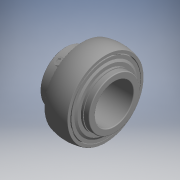
# Autodesk Inventor part: YAR 206-2RF-39.710300320618 -bearing
Saved by Autodesk Inventor 2017.3 (Build 213256000, 256)
## iProperties
Part Number: YAR 206-2RF-39.710300320618 -bearing
Material: Generic
Catalog Web Link: www.cadenas.de
Description: ayf_001hc_hh_hy_bearing-Y-bearings
Vendor: SKF
Document SubType Name: Modeling
Designer: partserver
Manufacturer: SKF
Mass: 35.182 g
Surface Area: 305.499 cm^2
Volume: 35.182 cm^3
Density: 1 g/cm^3
Appearance: PSOLRGB-175-175-175
Category: PARTsolutions
Company: SKF
Title: YAR 206-2RF-39.710300320618 -bearing
Author: Cadenas PARTsolutions
Comments: Y-bearings
PSOL_IDENT_0: {$CADENAS_DATA\23d-libs\skf\bearings_units_and_housings\bearing_units\ball_bearing_units\y-units\y-b
PSOL_IDENT_1: earing_square_flanged_units_parts\ayf_001hc_hh_hy_bearing.prj},231 {VTYP=3D},{NB=YAR 206-2RF-39.7103
PSOL_IDENT_2: 00320618 -bearing},{LINA=YAR 206-2RF-39.710300320618 -bearing},{NN=ayf_001hc_hh_hy_bearing},{DATE=20
PSOL_IDENT_3: .08.2020 13:45:20},{GEOMDATE=29.07.2020 17:09:33},{VERSION=},{LINEID=1120},{WBVAR=},{WBNUMERIC=}  {N
PSOL_IDENT_4: B=YAR 206-2RF-39.710300320618 -bearing},{LINA=YAR 206-2RF-39.710300320618 -bearing},{KT=DUMMY},{PROD
PSOL_IDENT_5: UCTID=103003206},{DESIGNATION=YAR 206-2RF},{DD=30.0000},{D=62},{B=38.100},{C=18.000},{PITCH=46.000},
PSOL_IDENT_6: {DW=9.525},{FO=IEC_BBY_006},{DESIGN=ybrg1},{B1=MIN},{LM=Grub screw},{DES=Inner ring extended on both
PSOL_IDENT_7: sides},{PS=For agricultural applications},{MAT=},{SS=Multiple seals},{UNIT=Metric},{G=MIN},{DD1=39.
PSOL_IDENT_8: 70},{DD2=MIN},{DD3=MIN},{B3=0.000},{B4=MIN},{BB4=5.0},{R12=0.6},{R12X=0},{SS1=22.200},{NOTE=},{DG=MI
PSOL_IDENT_9: N},{E=5.100},{F=1.700},{RG=MIN},{LOAD1=19.500},{LOAD2=11.200},{LOAD3=0.475},{SPEED2=3800},{FF0=14},{
PSOL_IDENT_10: BF=1},{A15=500000},{A8=400000},{A4=300000},{BETA=1.62},{SBT1=0.415},{SBT2=},{RF1=0.00000039},{RF2=1.
PSOL_IDENT_11: 7},{SF1=0.00323},{SF2=36.5},{KZ=3.1},{II=1},{Z=9},{SG=VT307},{MASS=0.31},{G2=M6x0.75},{HEX=3.000},{R
PSOL_IDENT_12: TT=4},{MKIT=},{AS=},{TANGLE=},{SLEEVE=},{SRING=RIS 206 A},{FPC=RBC17_YBRG_001},{POPI=1},{NOUN=N020},
PSOL_IDENT_13: {NOUNDES=Ball bearing},{MOD=M200},{MODDES=Radial deep groove},{YZ=19.85},{PIM=YAR 206-2RF},{LNDD11=M
PSOL_IDENT_14: IN},{LUB3=0},{BZ=0.565},{SDALG=h},{YRZ=27.7625},{SHAPE=5},{LNB1HM11=0},{LWM=0},{TYPEID=103003},{LUBG
PSOL_IDENT_15: R2=0},{LOCKNUT=},{LOCKDEVICE=},{LNB=MIN},{BB=MIN},{LNB1=MIN},{S1ALG=22.2},{HH=MIN},{LDB=MIN},{LDDD1=
PSOL_IDENT_16: MIN},{LDDD2=MIN},{LDM=MIN},{LDFF=MIN},{TP=4},{LNBHM11=0},{BBHM11=0},{LNDD1HM11=0},{HELP=5},{HHHM11=0
PSOL_IDENT_17: },{LUBGR1=0},{LWV=0},{S2=28.5},{LUB2=1},{BZ1=0.000},{HEX2=}
NB: YAR 206-2RF-39.710300320618 -bearing
NN: ayf_001hc_hh_hy_bearing
NT: Y-bearings
NBSYN: $DESIGNATION.-$DD1.$PRODUCTID.$C.$B1.-bearing
LINA: YAR 206-2RF-39.710300320618 -bearing
CATALOG: SKF
DESIGNATION: YAR 206-2RF
DD: 30
D: 62
B: 38.1
C: 18
B1: 0
DD1: 39.7
LOAD1: 19.5
LOAD2: 11.2
LOAD3: 0.475
SPEED2: 3800
SUPPLIER: SKF
ARTICLENO: YAR 206-2RF-39.710300320618 -bearing
BOMINFO: YAR 206-2RF-39.710300320618 -bearing
CREATOR: CADENAS GmbH
Autodesk Inventor part; units mm, degrees
sketch "Sketch_1" plane through (0, 0, 0) normal (0, 0, 1) x (1, 0, 0)
  line L0 (50, 0) -> (-50, 0)
  arc A0 (-15.9, 15.6) -> (-15.3, 15) centre (-15.3, 15.6) ccw
  line L1 (-15.3, 15) -> (21.6, 15)
  arc A1 (21.6, 15) -> (22.2, 15.6) centre (21.6, 15.6) ccw
  line L2 (22.2, 15.6) -> (22.2, 19.25)
  arc A2 (22.2, 19.25) -> (21.6, 19.85) centre (21.6, 19.25) ccw
  line L3 (21.6, 19.85) -> (3.572, 19.85)
  arc A3 (-3.572, 19.85) -> (3.572, 19.85) centre (0, 23) ccw
  line L4 (-3.572, 19.85) -> (-15.3, 19.85)
  arc A4 (-15.3, 19.85) -> (-15.9, 19.25) centre (-15.3, 19.25) ccw
  line L5 (-15.9, 19.25) -> (-15.9, 15.6)
  constraints: 12 end point, 10 point on circle, 5 centre point
revolve "Revolution1" add sketch "Sketch_1" angle 360 about axis through (50, 0, 0) along (1, 0, 0)
sketch "Sketch_2" plane through (0, 15, 0) normal (0, 1, 0) x (1, 0, 0)
  circle A0 centre (17.2, 0) radius 3
  line L0 (15.7, -0.866) -> (17.2, -1.7321)
  line L1 (17.2, -1.7321) -> (18.7, -0.866)
  line L2 (18.7, -0.866) -> (18.7, 0.866)
  line L3 (18.7, 0.866) -> (17.2, 1.7321)
  line L4 (17.2, 1.7321) -> (15.7, 0.866)
  line L5 (15.7, 0.866) -> (15.7, -0.866)
  constraints: 12 end point, 1 centre point
extrude "Extrusion1" add sketch "Sketch_2" along normal blind 5.335
sketch "Sketch_3" plane through (0, -7.5, -12.9904) normal (0, -0.5, -0.866) x (1, 0, 0)
  circle A0 centre (17.2, 0) radius 3
  line L0 (15.7, -0.866) -> (17.2, -1.7321)
  line L1 (17.2, -1.7321) -> (18.7, -0.866)
  line L2 (18.7, -0.866) -> (18.7, 0.866)
  line L3 (18.7, 0.866) -> (17.2, 1.7321)
  line L4 (17.2, 1.7321) -> (15.7, 0.866)
  line L5 (15.7, 0.866) -> (15.7, -0.866)
  constraints: 12 end point, 1 centre point
extrude "Extrusion2" add sketch "Sketch_3" along normal blind 5.335
sketch "Sketch_10" plane through (0, 0, 0) normal (0, 0, 1) x (1, 0, 0)
  line L0 (9, 0) -> (-9, 0)
  line L1 (-11.8525, 20.415) -> (-11.8525, 19.85)
  line L2 (-11.8525, 19.85) -> (-9.5925, 19.85)
  line L3 (-9.5925, 19.85) -> (-9.5925, 22.4564)
  arc A0 (-9.1678, 23.3393) -> (-9.5925, 22.4564) centre (-8.4625, 22.4564) ccw
  line L4 (-9.1678, 23.3393) -> (-8.435, 23.9246)
  line L5 (-8.435, 23.9246) -> (-8.435, 20.3248)
  line L6 (-8.435, 20.3248) -> (-7.87, 20.3248)
  line L7 (-7.87, 20.3248) -> (-7.87, 23.6289)
  line L8 (-7.87, 23.6289) -> (-6.0852, 24.8663)
  line L9 (-6.0852, 24.8663) -> (-6.0209, 24.7734)
  line L10 (-6.0209, 24.7734) -> (-7.757, 23.5697)
  line L11 (-7.757, 23.5697) -> (-7.757, 20.5621)
  line L12 (-7.757, 20.5621) -> (-6.1938, 20.5621)
  line L13 (-6.1938, 20.5621) -> (-6.3633, 19.85)
  line L14 (-6.3633, 19.85) -> (-5.7983, 19.85)
  line L15 (-5.7983, 19.85) -> (-5.61, 20.6413)
  line L16 (-5.61, 20.6413) -> (-5.61, 21.4325)
  line L17 (-5.61, 21.4325) -> (-6.3633, 22.2237)
  line L18 (-6.3633, 22.2237) -> (-6.3633, 23.8062)
  line L19 (-6.3633, 23.8062) -> (-5.61, 24.5975)
  line L20 (-5.61, 24.5975) -> (-5.61, 27.5742)
  arc A1 (-5.61, 27.5742) -> (-5.7983, 27.7625) centre (-5.7983, 27.5742) ccw
  line L21 (-5.7983, 27.7625) -> (-5.9867, 27.7625)
  arc A2 (-5.9867, 27.7625) -> (-6.175, 27.5742) centre (-5.9867, 27.5742) ccw
  line L22 (-6.175, 27.5742) -> (-7.1728, 26.385)
  line L23 (-7.1728, 26.385) -> (-6.74, 26.0218)
  line L24 (-6.74, 26.0218) -> (-6.175, 26.6952)
  line L25 (-6.175, 26.6952) -> (-6.175, 25.4916)
  line L26 (-6.175, 25.4916) -> (-7.6697, 24.4552)
  line L27 (-7.6697, 24.4552) -> (-8.7175, 24.5875)
  line L28 (-8.7175, 24.5875) -> (-8.7175, 26.98)
  line L29 (-8.7175, 26.98) -> (-9.2825, 26.98)
  line L30 (-9.2825, 26.98) -> (-9.2825, 24.5875)
  line L31 (-9.2825, 24.5875) -> (-10.1575, 23)
  line L32 (-10.1575, 23) -> (-10.1575, 20.415)
  line L33 (-10.1575, 20.415) -> (-11.8525, 20.415)
  constraints: 68 end point, 6 point on circle, 3 centre point
sketch "Sketch_15" plane through (0, 0, 0) normal (0, 0, 1) x (1, 0, 0)
  line L0 (9, 0) -> (-9, 0)
  line L1 (5.61, 27.5742) -> (5.61, 24.5975)
  line L2 (5.61, 24.5975) -> (6.3633, 23.8062)
  line L3 (6.3633, 23.8062) -> (6.3633, 22.2237)
  line L4 (6.3633, 22.2237) -> (5.61, 21.4325)
  line L5 (5.61, 21.4325) -> (5.61, 20.6413)
  line L6 (5.61, 20.6413) -> (5.7983, 19.85)
  line L7 (5.7983, 19.85) -> (6.3633, 19.85)
  line L8 (6.3633, 19.85) -> (6.1938, 20.5621)
  line L9 (6.1938, 20.5621) -> (7.757, 20.5621)
  line L10 (7.757, 20.5621) -> (7.757, 23.5697)
  line L11 (7.757, 23.5697) -> (6.0209, 24.7734)
  line L12 (6.0209, 24.7734) -> (6.0852, 24.8663)
  line L13 (6.0852, 24.8663) -> (7.87, 23.6289)
  line L14 (7.87, 23.6289) -> (7.87, 20.3248)
  line L15 (7.87, 20.3248) -> (8.435, 20.3248)
  line L16 (8.435, 20.3248) -> (8.435, 23.9246)
  line L17 (8.435, 23.9246) -> (9.1678, 23.3393)
  arc A0 (9.5925, 22.4564) -> (9.1678, 23.3393) centre (8.4625, 22.4564) ccw
  line L18 (9.5925, 22.4564) -> (9.5925, 19.85)
  line L19 (9.5925, 19.85) -> (11.8525, 19.85)
  line L20 (11.8525, 19.85) -> (11.8525, 20.415)
  line L21 (11.8525, 20.415) -> (10.1575, 20.415)
  line L22 (10.1575, 20.415) -> (10.1575, 23)
  line L23 (10.1575, 23) -> (9.2825, 24.5875)
  line L24 (9.2825, 24.5875) -> (9.2825, 26.98)
  line L25 (9.2825, 26.98) -> (8.7175, 26.98)
  line L26 (8.7175, 26.98) -> (8.7175, 24.5875)
  line L27 (8.7175, 24.5875) -> (7.6697, 24.4552)
  line L28 (7.6697, 24.4552) -> (6.175, 25.4916)
  line L29 (6.175, 25.4916) -> (6.175, 26.6952)
  line L30 (6.175, 26.6952) -> (6.74, 26.0218)
  line L31 (6.74, 26.0218) -> (7.1728, 26.385)
  line L32 (7.1728, 26.385) -> (6.175, 27.5742)
  arc A1 (6.175, 27.5742) -> (5.9867, 27.7625) centre (5.9867, 27.5742) ccw
  line L33 (5.9867, 27.7625) -> (5.7983, 27.7625)
  arc A2 (5.7983, 27.7625) -> (5.61, 27.5742) centre (5.7983, 27.5742) ccw
  constraints: 68 end point, 6 point on circle, 3 centre point
sketch "Sketch_16" plane through (0, 0, 0) normal (0, 0, 1) x (1, 0, 0)
  line L0 (9, 0) -> (-9, 0)
  line L1 (-9, 27.505) -> (-6.2842, 27.505)
  line L2 (-6.2842, 27.505) -> (-6.0901, 27.6774)
  arc A0 (-5.6026, 27.5218) -> (-6.0901, 27.6774) centre (-5.8925, 27.455) ccw
  line L3 (-5.6026, 27.5218) -> (-5.4743, 26.9651)
  arc A1 (-5.4743, 26.9651) -> (-5.2794, 26.81) centre (-5.2794, 27.01) ccw
  line L4 (-5.2794, 26.81) -> (-2.9409, 26.81)
  arc A2 (-2.9409, 26.81) -> (-2.792, 26.8582) centre (-2.9409, 27.064) ccw
  arc A3 (2.792, 26.8582) -> (-2.792, 26.8582) centre (0, 23) ccw
  arc A4 (2.792, 26.8582) -> (2.9409, 26.81) centre (2.9409, 27.064) ccw
  line L5 (2.9409, 26.81) -> (5.2794, 26.81)
  arc A5 (5.2794, 26.81) -> (5.4743, 26.9651) centre (5.2794, 27.01) ccw
  line L6 (5.4743, 26.9651) -> (5.6026, 27.5218)
  arc A6 (6.0901, 27.6774) -> (5.6026, 27.5218) centre (5.8925, 27.455) ccw
  line L7 (6.0901, 27.6774) -> (6.2842, 27.505)
  line L8 (6.2842, 27.505) -> (9, 27.505)
  line L9 (9, 27.505) -> (9, 29.5161)
  arc A7 (9, 29.5161) -> (8.8571, 29.7078) centre (8.8, 29.5161) ccw
  arc A8 (8.8571, 29.7078) -> (-8.8571, 29.7078) centre (0, 0) ccw
  arc A9 (-8.8571, 29.7078) -> (-9, 29.5161) centre (-8.8, 29.5161) ccw
  line L10 (-9, 29.5161) -> (-9, 27.505)
  constraints: 22 end point, 20 point on circle, 10 centre point
revolve "Revolution2" add sketch "Sketch_15" angle 360 about axis through (9, 0, 0) along (1, 0, 0)
revolve "Revolution3" add sketch "Sketch_16" angle 360 about axis through (9, 0, 0) along (1, 0, 0)
revolve "Revolution4" add sketch "Sketch_10" angle 360 about axis through (9, 0, 0) along (1, 0, 0)
sketch "Sketch_21" plane through (0, 0, 0) normal (0, 0, 1) x (1, 0, 0)
  line L0 (-4.1475, 23) -> (-4.1475, 46)
  line L1 (-4.1475, 46) -> (-3.2975, 46)
  line L2 (-3.2975, 46) -> (-3.2975, 23)
  line L3 (-3.2975, 23) -> (-4.1475, 23)
  line L4 (-4.1475, 23) -> (-4.1475, 46)
  constraints: 10 end point
revolve "Revolution5" cut sketch "Sketch_21" angle 360 about axis through (-4.1475, 23, 0) along (0, -1, 0)
ref_plane "ball_1_XY" through (0, 23, 0) normal (1, 0, 0) x (0, 0, -1)
ref_plane "ball_1_YZ" through (0, 23, 0) normal (0, 0, -1) x (0, 1, 0)
ref_plane "ball_1_ZX" through (0, 23, 0) normal (0, 1, 0) x (1, 0, 0)
ref_plane "ball_2_XY" through (0, 17.619, 14.7841) normal (1, 0, 0) x (0, 0, -1)
ref_plane "ball_2_YZ" through (0, 17.619, 14.7841) normal (0, 0, -1) x (0, 1, 0)
ref_plane "ball_2_ZX" through (0, 17.619, 14.7841) normal (0, 1, 0) x (1, 0, 0)
ref_plane "ball_3_XY" through (0, 3.9939, 22.6506) normal (1, 0, 0) x (0, 0, -1)
ref_plane "ball_3_YZ" through (0, 3.9939, 22.6506) normal (0, 0, -1) x (0, 1, 0)
ref_plane "ball_3_ZX" through (0, 3.9939, 22.6506) normal (0, 1, 0) x (1, 0, 0)
ref_plane "ball_4_XY" through (0, -11.5, 19.9186) normal (1, 0, 0) x (0, 0, -1)
ref_plane "ball_4_YZ" through (0, -11.5, 19.9186) normal (0, 0, -1) x (0, 1, 0)
ref_plane "ball_4_ZX" through (0, -11.5, 19.9186) normal (0, 1, 0) x (1, 0, 0)
ref_plane "ball_5_XY" through (0, -21.6129, 7.8665) normal (1, 0, 0) x (0, 0, -1)
ref_plane "ball_5_YZ" through (0, -21.6129, 7.8665) normal (0, 0, -1) x (0, 1, 0)
ref_plane "ball_5_ZX" through (0, -21.6129, 7.8665) normal (0, 1, 0) x (1, 0, 0)
ref_plane "ball_6_XY" through (0, -21.6129, -7.8665) normal (1, 0, 0) x (0, 0, -1)
ref_plane "ball_6_YZ" through (0, -21.6129, -7.8665) normal (0, 0, -1) x (0, 1, 0)
ref_plane "ball_6_ZX" through (0, -21.6129, -7.8665) normal (0, 1, 0) x (1, 0, 0)
ref_plane "ball_7_XY" through (0, -11.5, -19.9186) normal (1, 0, 0) x (0, 0, -1)
ref_plane "ball_7_YZ" through (0, -11.5, -19.9186) normal (0, 0, -1) x (0, 1, 0)
ref_plane "ball_7_ZX" through (0, -11.5, -19.9186) normal (0, 1, 0) x (1, 0, 0)
ref_plane "ball_8_XY" through (0, 3.9939, -22.6506) normal (1, 0, 0) x (0, 0, -1)
ref_plane "ball_8_YZ" through (0, 3.9939, -22.6506) normal (0, 0, -1) x (0, 1, 0)
ref_plane "ball_8_ZX" through (0, 3.9939, -22.6506) normal (0, 1, 0) x (1, 0, 0)
ref_plane "ball_9_XY" through (0, 17.619, -14.7841) normal (1, 0, 0) x (0, 0, -1)
ref_plane "ball_9_YZ" through (0, 17.619, -14.7841) normal (0, 0, -1) x (0, 1, 0)
ref_plane "ball_9_ZX" through (0, 17.619, -14.7841) normal (0, 1, 0) x (1, 0, 0)
ref_plane "brg_XY" through (0, 0, 0) normal (1, 0, 0) x (0, 0, -1)
ref_plane "brg_YZ" through (0, 0, 0) normal (0, 0, -1) x (0, 1, 0)
ref_plane "brg_ZX" through (0, 0, 0) normal (0, 1, 0) x (1, 0, 0)
ref_plane "brg3_XY" through (22.2, 0, 0) normal (1, 0, 0) x (0, 0, -1)
ref_plane "brg3_YZ" through (22.2, 0, 0) normal (0, 0, -1) x (0, 1, 0)
ref_plane "brg3_ZX" through (22.2, 0, 0) normal (0, 1, 0) x (1, 0, 0)
body "Solid1"
